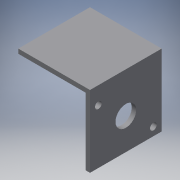
# Autodesk Inventor part: bag motor bracket
Saved by Autodesk Inventor 2016 (Build 200138000, 138)
## iProperties
Created: 2016-02-17
Part Number: bag motor bracket
Material: Generic
Document SubType Name: Modeling
Designer: gus
Density: 1 g/cm^3
Appearance: Default
Author: gus
Autodesk Inventor part; units mm, degrees
ref_plane "YZ Plane" through (0, 0, 0) normal (1, 0, 0) x (0, 1, 0)
ref_plane "XZ Plane" through (0, 0, 0) normal (0, 1, 0) x (-1, 0, 0)
ref_plane "XY Plane" through (0, 0, 0) normal (0, 0, 1) x (1, 0, 0)
sketch "Sketch1" plane through (0, 0, 0) normal (0, 0, 1) x (1, 0, 0)
  line L0 (0, 0) -> (0, -50.8)
  line L1 (0, -50.8) -> (-3.175, -50.8)
  line L2 (-3.175, -50.8) -> (-3.175, -3.175)
  line L3 (-3.175, -3.175) -> (-50.8, -3.175)
  line L4 (-50.8, -3.175) -> (-50.8, 0)
  line L5 (-50.8, 0) -> (0, 0)
  dimension "d0" = 50.8
  dimension "d1" = 3.175
  dimension "d2" = 47.625
  dimension "d3" = 47.625
  constraints: 12 end point, 5 perpendicular, 1 vertical
  measures "d0" distance of L0.start L0.end
  measures "d1" distance of L0.end L1.end
  measures "d2" distance of L1.end L2.end
  measures "d3" distance of L2.end L3.end
extrude "Extrusion1" add sketch "Sketch1" along normal blind 50.8
sketch "Sketch2" plane through (-3.175, -50.8, 0) normal (-1, 0, 0) x (0, 0, 1)
  circle A0 centre (25.4, 22.225) radius 9.525
  line L0 (0, 50.8) -> (0, 0) projected
  line L1 (0, 0) -> (50.8, 0) projected
  circle A1 centre (25.4, 22.225) radius 25.4 construction
  circle A2 centre (44.8818, 38.5228) radius 2.3813
  circle A3 centre (5.9223, 5.9223) radius 2.3813
  line L2 (5.9223, 5.9223) -> (5.9223, 50.8) construction
  line L3 (0, 50.8) -> (50.8, 50.8) construction
  line L4 (5.9223, 5.9223) -> (0, 5.9223) construction
  line L5 (5.9223, 5.9223) -> (5.9223, 0) construction
  line L6 (50.8, 0) -> (50.8, 50.8) construction
  dimension "d9" = 25.4
  dimension "d10" = 22.225
  dimension "d13" = 50.8
  dimension "d14" = 4.7625
  dimension "d15" = 4.7625
  dimension "d16" = 5.9182
  dimension "d17" = 19.05
  constraints: 6 end point, 4 centre point, 3 perpendicular, 3 point on line, 2 coincident, 2 point on circle, 1 vertical
  measures "d9" distance from line of L0 A0.centre
  measures "d10" distance from line of L1 A0.centre
  measures "d13" diameter of A1
  measures "d14" diameter of A2
  measures "d15" diameter of A3
  measures "d16" distance from line of L6 A2.centre
  measures "d17" diameter of A0
extrude "Extrusion2" cut sketch "Sketch2" against normal blind 3.175
body "Solid1"
